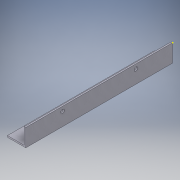
# Autodesk Inventor part: new  L clamp
Saved by Autodesk Inventor 2019 (Build 230136000, 136)
## iProperties
Created: 2020-02-29
Part Number: new  L clamp
Material: Stainless Steel AISI 440C, Welded
Document SubType Name: Modeling
Designer: KiranM
Density: 7.8 g/cm^3
Appearance: Weld - Stainless Steel
Author: KiranM
Autodesk Inventor part; units mm, degrees
ref_plane "YZ Plane" through (0, 0, 0) normal (1, 0, 0) x (0, 1, 0)
ref_plane "XZ Plane" through (0, 0, 0) normal (0, 1, 0) x (-1, 0, 0)
ref_plane "XY Plane" through (0, 0, 0) normal (0, 0, 1) x (1, 0, 0)
sketch "Sketch1" plane through (0, 0, 0) normal (0, 0, 1) x (1, 0, 0)
  line L0 (0, 0) -> (0, -24)
  line L1 (0, -24) -> (-25, -24)
  line L2 (-25, -24) -> (-25, -22)
  line L3 (0, 0) -> (-2, 0)
  line L4 (-2, 0) -> (-2, -22)
  line L5 (-2, -22) -> (-25, -22)
  constraints: 12 end point, 4 perpendicular, 1 horizontal, 1 vertical
extrude "Extrusion1" add sketch "Sketch1" along normal blind 200
sketch "Sketch2" plane through (-2, -22, 0) normal (-1, 0, 0) x (0, 0, 1)
  circle A0 centre (50, 16) radius 2.5
  circle A1 centre (150, 16) radius 2.5
  point P0 (200, 22)
  constraints: 2 centre point
extrude "Extrusion2" cut sketch "Sketch2" against normal through all
sketch "Sketch3" plane through (0, -24, 0) normal (1, 0, 0) x (0, 0, -1)
  point P0 (0, 24)
body "Solid1"
